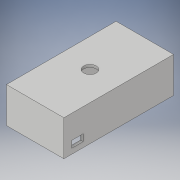
# Autodesk Inventor part: 호출벨 new
Saved by Autodesk Inventor 2019.5 (Build 235369000, 369)
## iProperties
Created: 2021-08-25
Part Number: 호출벨 new
Material: 일반
Document SubType Name: Modeling
Designer: msj19
Density: 1 g/cm^3
Appearance: 기본값
Author: msj19
Autodesk Inventor part; units mm, degrees
ref_plane "우측면도" through (0, 0, 0) normal (1, 0, 0) x (0, 1, 0)
ref_plane "평면도" through (0, 0, 0) normal (0, 1, 0) x (-1, 0, 0)
ref_plane "정면도" through (0, 0, 0) normal (0, 0, 1) x (1, 0, 0)
sketch "스케치1" plane through (0, 0, 0) normal (0, 1, 0) x (-1, 0, 0)
  line L0 (0, 0) -> (0, -100)
  line L1 (0, -100) -> (-50, -100)
  line L2 (-50, -100) -> (-50, 0)
  line L3 (-50, 0) -> (0, 0)
  line L4 (2.5, -102.5) -> (2.5, 2.5)
  line L5 (2.5, 2.5) -> (-52.5, 2.5)
  line L6 (-52.5, 2.5) -> (-52.5, -102.5)
  line L7 (-52.5, -102.5) -> (2.5, -102.5)
  line L8 (1, -101) -> (1, 1)
  line L9 (1, 1) -> (-51, 1)
  line L10 (-51, 1) -> (-51, -101)
  line L11 (-51, -101) -> (1, -101)
  line L12 (1.5, -101.5) -> (1.5, 1.5)
  line L13 (1.5, 1.5) -> (-51.5, 1.5)
  line L14 (-51.5, 1.5) -> (-51.5, -101.5)
  line L15 (-51.5, -101.5) -> (1.5, -101.5)
  dimension "d1" = 50
  dimension "d2" = 100
  dimension "d5" = 2.5
  dimension "d6" = 1.5
  dimension "d7" = 0.5
  constraints: 32 end point, 12 perpendicular, 1 vertical, 9 other
  measures "d1" distance between parallel lines of L2 L0
  measures "d2" distance between parallel lines of L3 L1
  measures "d5" distance between parallel lines of L0 L4
  measures "d6" distance between parallel lines of L0 L12
  measures "d7" distance between parallel lines of L12 L8
extrude "돌출1" add sketch "스케치1" along normal blind 34 contours L7 L6 L5 L4 | L11 L10 L9 L8 | L15 L14 L13 L12
sketch "스케치4" plane through (50, 0, 0) normal (-1, 0, 0) x (0, 0, 1)
  line L0 (-100, 34) -> (0, 34) projected
  line L1 (-100, 34) -> (0, 34)
  line L2 (0, 34) -> (0, 31.5)
  line L3 (0, 31.5) -> (-100, 31.5)
  line L4 (-100, 34) -> (-100, 31.5)
  line L5 (0, 34) -> (0, 31.5)
  point P0 (0, 0)
  dimension "d12" = 2.5
  constraints: 10 end point, 2 collinear, 2 vertical, 1 perpendicular
  measures "d12" distance between parallel lines of L3 L0
sketch "스케치5" plane through (0, 0, -100) normal (1, 0, 0) x (0, 0, -1)
  line L0 (-100, 34) -> (0, 34) projected
  line L1 (0, 34) -> (0, 31.5)
  line L2 (0, 31.5) -> (-100, 31.5)
  line L3 (-100, 34) -> (-100, 31.5)
  line L4 (-100, 34) -> (0, 34)
  point P0 (-100, 0)
  dimension "d13" = 2.5
  constraints: 8 end point, 2 perpendicular, 2 vertical
  measures "d13" distance between parallel lines of L2 L0
loft "로프트1" add profiles "스케치4", "스케치5"
sketch "스케치6" plane through (0, 34, 0) normal (0, 1, 0) x (1, 0, 0)
  line L0 (-2.5, 102.5) -> (-2.5, -2.5) projected
  line L1 (-2.5, -2.5) -> (52.5, -2.5) projected
  line L2 (52.5, -2.5) -> (52.5, 102.5) projected
  line L3 (52.5, 102.5) -> (-2.5, 102.5) projected
  circle A0 centre (25, 50) radius 6
  point P0 (0, 0)
  dimension "d18" = 12
  dimension "d31" = 27.5
  dimension "d32" = 52.5
  constraints: 1 centre point
  measures "d18" diameter of A0
  measures "d31" distance from line of L0 A0.centre
  measures "d32" distance from line of L3 A0.centre
extrude "돌출2" cut sketch "스케치6" against normal blind 50 contours A0
sketch "스케치8" plane through (0, 0, 0) normal (0, -1, 0) x (1, 0, 0)
  line L0 (50, -100) -> (0, -100) projected
  line L1 (0, -100) -> (0, 0) projected
  line L2 (0, 0) -> (50, 0) projected
  line L3 (50, 0) -> (50, -100) projected
  line L4 (-2.5, -102.5) -> (-2.5, 2.5) projected
  line L5 (52.5, -102.5) -> (-2.5, -102.5) projected
  line L6 (52.5, 2.5) -> (52.5, -102.5) projected
  line L7 (-2.5, 2.5) -> (52.5, 2.5) projected
  line L8 (-1.5, -101.5) -> (-1.5, 1.5) projected
  line L9 (-1, -101) -> (-1, 1) projected
  line L10 (-1.5, 1.5) -> (51.5, 1.5) projected
  line L11 (-1, 1) -> (51, 1) projected
  line L12 (51, 1) -> (51, -101) projected
  line L13 (51.5, 1.5) -> (51.5, -101.5) projected
  line L14 (51, -101) -> (-1, -101) projected
  line L15 (51.5, -101.5) -> (-1.5, -101.5) projected
extrude "돌출4" cut sketch "스케치8" against normal blind 2.5 contours L8 L10 L13 L15
sketch "스케치9" plane through (52.5, 0, 2.5) normal (1, 0, 0) x (0, 0, -1)
  line L0 (0, 0) -> (105, 0) projected
  line L1 (105, 0) -> (105, 34) projected
  line L2 (0, 34) -> (105, 34) projected
  line L3 (0, 0) -> (0, 34) projected
  line L4 (7.5, 11.5) -> (18.5, 11.5)
  line L5 (18.5, 11.5) -> (18.5, 5)
  line L6 (18.5, 5) -> (7.5, 5)
  line L7 (7.5, 5) -> (7.5, 11.5)
  point P0 (2.5, 0)
  dimension "d25" = 6.5
  dimension "d26" = 11
  dimension "d27" = 5
  dimension "d28" = 5
  constraints: 8 end point, 2 parallel, 1 horizontal, 1 perpendicular
  measures "d25" distance between parallel lines of L6 L4
  measures "d26" distance between parallel lines of L5 L7
  measures "d27" distance from line of point (2.5, 0) L7
  measures "d28" distance between parallel lines of L0 L6
extrude "돌출5" cut sketch "스케치9" against normal blind 10 contours L4 L5 L6 L7
